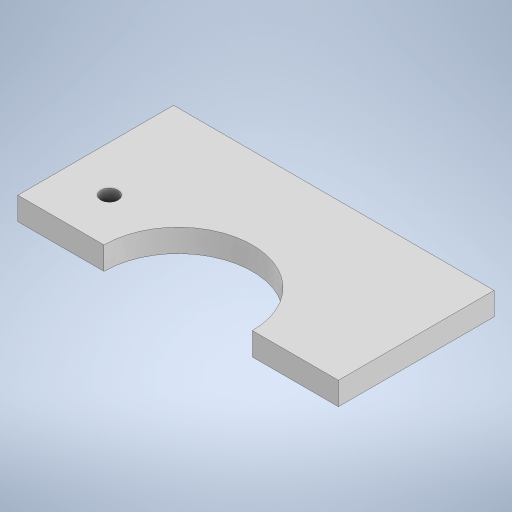
# Autodesk Inventor part: sguard
Saved by Autodesk Inventor 2023 (Build 270158000, 158)
## iProperties
Created: 2023-03-16
Part Number: sguard
Material: Generic
Document SubType Name: Modeling
Designer: ianjo
Density: 1 g/cm^3
Appearance: Default
Author: ianjo
Autodesk Inventor part; units mm, degrees
ref_plane "YZ Plane" through (0, 0, 0) normal (1, 0, 0) x (0, 1, 0)
ref_plane "XZ Plane" through (0, 0, 0) normal (0, 1, 0) x (-1, 0, 0)
ref_plane "XY Plane" through (0, 0, 0) normal (0, 0, 1) x (1, 0, 0)
sketch "Sketch1" plane through (0, 0, 0) normal (0, 1, 0) x (-1, 0, 0)
  line L0 (-44.45, 21.59) -> (44.45, 21.59)
  line L1 (44.45, 21.59) -> (44.45, -21.59)
  line L2 (44.45, -21.59) -> (-44.45, -21.59)
  line L3 (-44.45, -21.59) -> (-44.45, 21.59)
  line L4 (-44.45, 21.59) -> (44.45, -21.59) construction
  line L5 (44.45, 21.59) -> (-44.45, -21.59) construction
  point P0 (0, 0)
  dimension "d5" = 88.9
  dimension "d6" = 43.18
  constraints: 12 end point, 2 midpoint, 2 parallel, 1 horizontal, 1 perpendicular
  measures "d5" distance of L1.end L2.end
  measures "d6" distance of L0.end L1.end
extrude "Extrusion1" add sketch "Sketch1" along normal blind 6.35
sketch "Sketch2" plane through (0, 6.35, 0) normal (0, 1, 0) x (1, 0, 0)
  line L0 (44.45, 21.59) -> (-44.45, 21.59) projected
  line L1 (44.45, -21.59) -> (44.45, 21.59) projected
  point P0 (0, 0)
  point P1 (0, -21.59)
  dimension "d16" = 43.18
  dimension "d17" = 44.45
  measures "d16" distance from line of L0 point (0, -21.59)
  measures "d17" distance from line of L1 point (0, -21.59)
hole "Hole1" at (0, 6.35, 21.59) direction (0, -1, 0) diameter 41.148 end through all
sketch "Sketch3" plane through (0, 6.35, 0) normal (0, 1, 0) x (1, 0, 0)
  line L0 (-44.45, 21.59) -> (-44.45, -21.59) projected
  line L1 (-44.45, -21.59) -> (-20.574, -21.59) projected
  point P0 (0, 0)
  point P1 (-31.75, -8.89)
  dimension "d25" = 12.7
  dimension "d26" = 12.7
  measures "d25" distance from line of L0 point (-31.75, -8.89)
  measures "d26" distance from line of L1 point (-31.75, -8.89)
hole "Hole2" at (-31.75, 6.35, 8.89) direction (0, -1, 0) diameter 4.826 end through all
body "Solid1"
